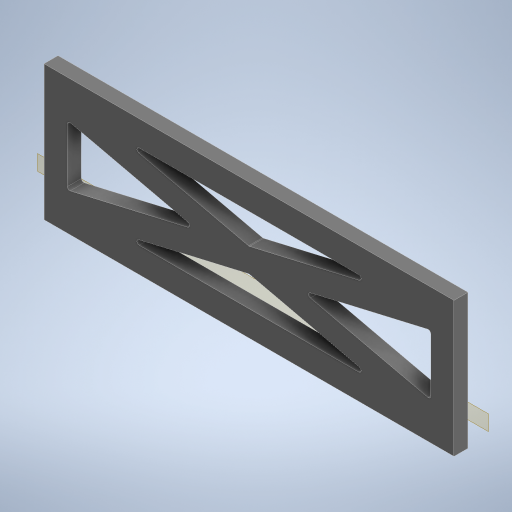
# Autodesk Inventor part: 13
Saved by Autodesk Inventor 2024.3 (Build 283343000, 343)
## iProperties
Created: 2024-09-08
Part Number: 13
Material: 아크릴, 선명
Document SubType Name: Modeling
Designer: 구지현
Density: 1.19 g/cm^3
Appearance: 회색
Mass: 52.1703 g
Surface Area: 217.666 cm^2
Volume: 43.8406 cm^3
Author: 구지현
Autodesk Inventor part; units mm, degrees
ref_plane "YZ Plane" through (0, 0, 0) normal (1, 0, 0) x (0, 1, 0)
ref_plane "XZ Plane" through (0, 0, 0) normal (0, 1, 0) x (-1, 0, 0)
ref_plane "XY Plane" through (0, 0, 0) normal (0, 0, 1) x (1, 0, 0)
ref_plane "작업 평면1" through (0, 0, 0) normal (0, 0, 1) x (1, 0, 0)
sketch "스케치1" plane through (0, 0, 0) normal (0, 0, 1) x (1, 0, 0)
  line L0 (0, 0) -> (176, 0) projected
  line L1 (176, 0) -> (176, 6) projected
  line L2 (0, 6) -> (176, 6) projected
  line L3 (0, 0) -> (0, 6) projected
  line L4 (0, 0) -> (176, 0)
  line L5 (176, 0) -> (176, 70)
  line L6 (176, 70) -> (0, 70)
  line L7 (0, 70) -> (0, 0)
  line L8 (0, 3) -> (25, 3)
  line L9 (25, 3) -> (25, 3)
  line L10 (25, 3) -> (0, 3)
  line L11 (0, 3) -> (0, 3)
  line L12 (25, 3) -> (67, 3)
  line L13 (67, 3) -> (109, 3)
  line L14 (109, 3) -> (151, 3)
  line L15 (151, 3) -> (176, 3)
  line L16 (151, 3) -> (151, 6)
  line L17 (151, 3) -> (151, 0)
  line L18 (109, 3) -> (109, 0)
  line L19 (109, 3) -> (109, 6)
  line L20 (67, 3) -> (67, 0)
  line L21 (67, 3) -> (67, 6)
  line L22 (25, 3) -> (25, 0)
  line L23 (25, 3) -> (25, 6)
  line L24 (0, 70) -> (0, 64)
  line L25 (0, 64) -> (176, 64)
  line L26 (25, 3) -> (25, 70)
  line L27 (67, 3) -> (67, 70)
  line L28 (109, 3) -> (109, 70)
  line L29 (151, 3) -> (151, 70)
  line L30 (20, 50) -> (156, 50)
  line L31 (156, 50) -> (156, 20)
  line L32 (156, 20) -> (18.9212, 20)
  line L33 (20, 50) -> (20, 20)
  point P0 (25, 0)
  point P1 (67, 0)
  point P2 (109, 0)
  point P3 (151, 0)
  point P4 (151, 64)
  point P5 (109, 64)
  point P6 (67, 64)
  point P7 (25, 64)
  point P8 (20, 38.5106)
  point P9 (76.3623, 50)
  point P10 (156, 43.8012)
  point P11 (88, 20)
  point P12 (151, 50)
  point P13 (151, 20)
  dimension "d0" = 176
  dimension "d1" = 70
  dimension "d2" = 25
  dimension "d3" = 42
  dimension "d4" = 42
  dimension "d5" = 42
  dimension "d6" = 25
  dimension "d7" = 6
  dimension "d10" = 20
  dimension "d11" = 20
  dimension "d12" = 20
  dimension "d13" = 20
  constraints: 60 end point, 22 point on line, 14 perpendicular, 5 equal length, 4 horizontal
  measures "d0" distance of L6.end L5.end
  measures "d1" distance of L5.end L4.end
  measures "d2" distance of L10.end L9.end
  measures "d3" distance of L8.end L12.end
  measures "d4" distance of L12.end L13.end
  measures "d5" distance of L13.end L14.end
  measures "d6" distance of L14.end L15.end
  measures "d7" distance of L6.end L24.end
  measures "d10" distance from line of L5 point (156, 43.801)
  measures "d11" distance from line of L6 point (76.362, 50)
  measures "d12" distance from line of L0 point (88, 20)
  measures "d13" distance from line of L7 point (20, 38.511)
extrude "돌출1" add sketch "스케치1" along normal blind 6 contours L3 L8 L22 L0 | L3 L2 L23 L8 | L20 L13 L18 L0 | L7 L25 L26 L30 L33 L32 L2 | L21 L2 L19 L13 | L26 L32 L27 L2 | L7 L6 L26 L25 | L17 L15 L1 L0 | L27 L32 L28 L2 | L25 L27 L30 L26 | L16 L2 L1 L15 | L28 L32 L29 L2 | L27 L6 L28 L25 | L25 L28 L30 L27 | L29 L32 L31 L30 L25 L5 L2 | L25 L29 L30 L28 | L29 L30 L31 L32 | L29 L6 L5 L25
move faces "이동1" translate (0, -10, 0) faces at (20, 30, 2) (107.3333, 20, 4) (151, 40, 4) (123, 6, 2) (159.3333, 0, 2) (81, 0, 4) (39, 6, 4) (8.3333, 0, 2) (25, 1, 2) (25, 4, 2) (109, 1, 2) (109, 4, 2) (67, 5, 2) (67, 2, 2) (151, 2, 2) (151, 5, 2)
sketch "스케치2" plane through (176, 70, 6) normal (1, 0, 0) x (0, 0, -1)
  line L0 (6, -60) -> (6, -74) projected
  line L1 (6, -74) -> (15, -74) projected
  line L2 (15, -74) -> (15, -80) projected
  line L3 (15, -80) -> (35, -80) projected
  line L4 (35, -80) -> (35, -74) projected
  line L5 (35, -74) -> (50, -74) projected
  line L6 (50, -74) -> (50, -80) projected
  line L7 (50, -80) -> (70, -80) projected
  line L8 (70, -80) -> (70, -74) projected
  line L9 (70, -74) -> (79, -74) projected
  line L10 (79, -74) -> (79, -60) projected
  line L11 (79, -60) -> (85, -60) projected
  line L12 (85, -60) -> (85, -20) projected
  line L13 (85, -20) -> (79, -20) projected
  line L14 (79, -20) -> (79, 0) projected
  line L15 (79, 0) -> (70, 0) projected
  line L16 (70, 0) -> (70, -6) projected
  line L17 (70, -6) -> (50, -6) projected
  line L18 (50, -6) -> (50, 0) projected
  line L19 (50, 0) -> (35, 0) projected
  line L20 (35, 0) -> (35, -6) projected
  line L21 (35, -6) -> (15, -6) projected
  line L22 (15, -6) -> (15, 0) projected
  line L23 (15, 0) -> (6, 0) projected
  line L24 (6, 0) -> (6, -20) projected
  line L25 (6, -20) -> (0, -20) projected
  line L26 (0, -20) -> (0, -60) projected
  line L27 (0, -60) -> (6, -60) projected
  line L28 (6, -80) -> (6, 0) projected
  line L29 (6, 0) -> (0, 0) projected
  line L30 (0, -80) -> (0, 0) projected
  line L31 (6, -80) -> (0, -80) projected
  point P0 (6, -70)
  point P1 (0, -60)
  point P2 (6, 0)
  point P3 (0, -20)
extrude "돌출2" cut sketch "스케치2" against normal blind 6 contours L28 L24 L23 L22 L21 L20 L19 L18 L17 L16 L15 L14 L13 L12 L11 L10 L9 L8 L7 L6 L5 L4 L3 L2 L1 L0 | L27 L26 L25 L28
sketch "스케치3" plane through (0, 70, 0) normal (-1, 0, 0) x (0, 0, 1)
  ellipse E0 centre (-18.9548, -43.9) end of major axis (-18.9548, -42.45) minor radius 1.45 projected
  ellipse E1 centre (-53.5548, -21.9) end of major axis (-53.5548, -20.45) minor radius 1.45 projected
  ellipse E2 centre (-18.9548, -65.9) end of major axis (-18.9548, -64.45) minor radius 1.45 projected
  circle A0 centre (-18.9548, -21.9) radius 1.45 projected
  circle A1 centre (-53.5548, -43.9) radius 1.45 projected
  ellipse E3 centre (-53.5548, -65.9) end of major axis (-53.5548, -64.45) minor radius 1.45 projected
  line L0 (-51.1548, -74) -> (-44, -74) projected
  line L1 (-44, -74) -> (-44, -80) projected
  line L2 (-44, -80) -> (-64, -80) projected
  line L3 (-64, -80) -> (-64, -74) projected
  line L4 (-64, -74) -> (-73, -74) projected
  line L5 (-73, -74) -> (-73, -60) projected
  line L6 (-73, -60) -> (-79, -60) projected
  line L7 (-79, -60) -> (-79, -20) projected
  line L8 (-79, -20) -> (-73, -20) projected
  line L9 (-73, -20) -> (-73, 0) projected
  line L10 (-73, 0) -> (-64, 0) projected
  line L11 (-64, 0) -> (-64, -6) projected
  line L12 (-64, -6) -> (-44, -6) projected
  line L13 (-44, -6) -> (-44, 0) projected
  line L14 (-44, 0) -> (-29, 0) projected
  line L15 (-29, 0) -> (-29, -6) projected
  line L16 (-29, -6) -> (-9, -6) projected
  line L17 (-9, -6) -> (-9, 0) projected
  line L18 (-9, 0) -> (0, 0) projected
  line L19 (0, 0) -> (0, -20) projected
  line L20 (0, -20) -> (6, -20) projected
  line L21 (6, -20) -> (6, -60) projected
  line L22 (6, -60) -> (0, -60) projected
  line L23 (0, -60) -> (0, -74) projected
  line L24 (0, -74) -> (-9, -74) projected
  line L25 (-9, -74) -> (-9, -80) projected
  line L26 (-9, -80) -> (-29, -80) projected
  line L27 (-29, -80) -> (-29, -74) projected
  line L28 (-29, -74) -> (-21.3548, -74) projected
  line L29 (-21.3548, -74) -> (-21.3548, -12.9525) projected
  line L30 (-21.3548, -12.9525) -> (-24.7548, -13) projected
  line L31 (-24.7548, -13) -> (-50.8207, -13) projected
  ellipse E4 centre (-50.1962, -14.9) end of major axis (-50.1962, -12.9) minor radius 2 (-50.8207, -13) -> (-50.8548, -13.0115) ccw projected
  line L32 (-50.8548, -13.0115) -> (-50.8548, -13) projected
  line L33 (-50.8548, -13) -> (-51.1548, -13) projected
  line L34 (-51.1548, -13) -> (-51.1548, -13.1447) projected
  ellipse E5 centre (-50.1962, -14.9) end of major axis (-50.1962, -16.9) minor radius 2 (-50.8548, -13.0115) -> (-51.1548, -13.1447) ccw projected
  line L35 (-50.8548, -13.0115) -> (-50.8548, -13.1178) projected
  arc A2 (-50.8548, -13.1178) -> (-51.1548, -13.2595) centre (-50.1963, -14.8999) ccw projected
  line L36 (-51.1548, -13.2595) -> (-51.1548, -74) projected
  line L37 (0, 0) -> (0, -80) projected
  line L38 (0, -80) -> (6, -80) projected
  line L39 (6, 0) -> (6, -80) projected
  line L40 (0, 0) -> (6, 0) projected
  point P0 (0, -70)
  point P1 (0, -20)
  point P2 (0, -60)
  constraints: 2 other
extrude "돌출3" cut sketch "스케치3" against normal blind 6 contours L37 L20 L21 L22
sketch "스케치4" plane through (0, 0, 6) normal (0, 0, 1) x (1, 0, 0)
  line L0 (54, 56) -> (20, 56) projected
  line L1 (20, 56) -> (20, 50) projected
  line L2 (20, 50) -> (54, 50) projected
  line L3 (54, 50) -> (54, 56) projected
  line L4 (117, 50) -> (151, 50) projected
  line L5 (151, 50) -> (151, 56) projected
  line L6 (151, 56) -> (117, 56) projected
  line L7 (117, 56) -> (117, 50) projected
  line L8 (117, 4) -> (151, 4) projected
  line L9 (151, 4) -> (151, 10) projected
  line L10 (151, 10) -> (117, 10) projected
  line L11 (117, 10) -> (117, 4) projected
  line L12 (54, 10) -> (20, 10) projected
  line L13 (20, 10) -> (20, 4) projected
  line L14 (20, 4) -> (54, 4) projected
  line L15 (54, 4) -> (54, 10) projected
  point P0 (0, 0)
extrude "돌출4" cut sketch "스케치4" against normal blind 6
sketch "스케치5" plane through (0, 0, 6) normal (0, 0, 1) x (1, 0, 0)
  line L0 (151, 56) -> (151, 10) projected
  line L1 (151, 10) -> (151, 4) projected
  line L2 (151, 4) -> (117, 4) projected
  line L3 (117, 4) -> (117, 10) projected
  line L4 (117, 10) -> (54, 10) projected
  line L5 (54, 10) -> (54, 4) projected
  line L6 (54, 4) -> (20, 4) projected
  line L7 (20, 4) -> (20, 56) projected
  line L8 (20, 56) -> (54, 56) projected
  line L9 (54, 56) -> (54, 50) projected
  line L10 (54, 50) -> (117, 50) projected
  line L11 (117, 50) -> (117, 56) projected
  line L12 (117, 56) -> (151, 56) projected
  line L13 (6, 10) -> (0, 10) projected
  line L14 (0, 10) -> (0, -10) projected
  line L15 (0, -10) -> (25, -10) projected
  line L16 (25, -10) -> (25, -4) projected
  line L17 (25, -4) -> (67, -4) projected
  line L18 (67, -4) -> (67, -10) projected
  line L19 (67, -10) -> (109, -10) projected
  line L20 (109, -10) -> (109, -4) projected
  line L21 (109, -4) -> (151, -4) projected
  line L22 (151, -4) -> (151, -10) projected
  line L23 (151, -10) -> (176, -10) projected
  line L24 (176, -10) -> (176, 10) projected
  line L25 (176, 10) -> (170, 10) projected
  line L26 (170, 10) -> (170, 50) projected
  line L27 (170, 50) -> (176, 50) projected
  line L28 (176, 50) -> (176, 70) projected
  line L29 (176, 70) -> (151, 70) projected
  line L30 (151, 70) -> (151, 64) projected
  line L31 (151, 64) -> (109, 64) projected
  line L32 (109, 64) -> (109, 70) projected
  line L33 (109, 70) -> (67, 70) projected
  line L34 (67, 70) -> (67, 64) projected
  line L35 (67, 64) -> (25, 64) projected
  line L36 (25, 64) -> (25, 70) projected
  line L37 (25, 70) -> (0, 70) projected
  line L38 (0, 70) -> (0, 50) projected
  line L39 (0, 50) -> (6, 50) projected
  line L40 (6, 50) -> (6, 10) projected
  line L41 (0, 70) -> (176, 70)
  line L42 (176, 70) -> (176, -10)
  line L43 (176, -10) -> (0, -10)
  line L44 (0, -10) -> (0, 70)
  point P0 (0, 0)
  point P1 (176, 50)
  point P2 (0, 10)
  point P3 (67, 70)
  constraints: 8 end point, 2 parallel, 1 horizontal, 1 perpendicular
extrude "돌출5" add sketch "스케치5" against normal up to surface (6 mm away) contours L0 L1 L2 L3 L4 L5 L6 L7 L8 L9 L10 L11 L12 | L13 L44 L39 L40 | L16 L17 L18 L43 | L41 L34 L35 L36 | L20 L21 L22 L43 | L41 L30 L31 L32 | L25 L26 L27 L42
sketch "스케치6" plane through (0, 0, 6) normal (0, 0, 1) x (1, 0, 0)
  line L0 (0, 70) -> (0, -10) projected
  line L1 (0, -10) -> (176, -10) projected
  line L2 (176, -10) -> (176, 70) projected
  line L3 (176, 70) -> (0, 70) projected
  line L4 (166, 0) -> (10, 0)
  line L5 (10, 0) -> (10, 60)
  line L6 (10, 60) -> (166, 60)
  line L7 (166, 60) -> (166, 0)
  line L8 (10, 60) -> (166, 0)
  line L9 (10, 0) -> (166, 60)
  line L10 (11.4359, 63.7334) -> (167.4359, 3.7334)
  line L11 (8.5641, 3.7334) -> (164.5641, 63.7334)
  line L12 (11.4359, -3.7334) -> (167.4359, 56.2666)
  line L13 (8.5641, 56.2666) -> (164.5641, -3.7334)
  point P0 (0, 0)
  point P1 (154.8573, 0)
  point P2 (88, 25.7143)
  point P3 (21.1427, 0)
  point P4 (166, 55.7143)
  point P5 (99.1427, 30)
  point P6 (166, 4.2857)
  point P7 (88, 34.2857)
  point P8 (154.8573, 60)
  point P9 (21.1427, 60)
  point P10 (76.8573, 30)
  point P11 (10, 55.7143)
  point P12 (10, 4.2857)
  dimension "d25" = 10
  dimension "d26" = 4
  dimension "d27" = 4
  dimension "d28" = 4
  dimension "d29" = 4
  constraints: 20 end point, 4 parallel, 3 other
  measures "d25" distance between parallel lines of L1 L4
  measures "d26" distance between parallel lines of L8 L10
  measures "d27" distance between parallel lines of L9 L11
  measures "d28" distance between parallel lines of L9 L12
  measures "d29" distance between parallel lines of L8 L13
extrude "돌출6" cut sketch "스케치6" against normal through all contours L4 L12 L13 | L10 L12 L7 | L5 L13 L11 | L11 L10 L6
fillet "모깎기1" radius 5 11 edges at (10, 55.7143, 3) (21.1427, 60, 3) (154.8573, 60, 3) (166, 55.7143, 3) (166, 4.2857, 3) (99.1427, 30, 3) (88, 34.2857, 3) (76.8573, 30, 3) (88, 25.7143, 3) (10, 4.2857, 3) (21.1427, 0, 3)
sketch "스케치7" plane through (0, 0, 0) normal (0, 0, -1) x (-1, 0, 0)
  line L0 (-166, 11.5658) -> (-166, 48.4342) projected
  arc A0 (-159.2051, 53.1009) -> (-166, 48.4342) centre (-161, 48.4342) ccw projected
  line L1 (-159.2051, 53.1009) -> (-111.2762, 34.6667) projected
  arc A1 (-111.2762, 25.3333) -> (-111.2762, 34.6667) centre (-113.0711, 30) ccw projected
  line L2 (-111.2762, 25.3333) -> (-159.2051, 6.8991) projected
  arc A2 (-166, 11.5658) -> (-159.2051, 6.8991) centre (-161, 11.5658) ccw projected
  line L3 (-46.2762, 50.3333) -> (-86.2051, 34.976) projected
  arc A3 (-89.7949, 34.976) -> (-86.2051, 34.976) centre (-88, 39.6427) ccw projected
  line L4 (-89.7949, 34.976) -> (-129.7238, 50.3333) projected
  arc A4 (-127.9289, 60) -> (-129.7238, 50.3333) centre (-127.9289, 55) ccw projected
  line L5 (-127.9289, 60) -> (-48.0711, 60) projected
  arc A5 (-46.2762, 50.3333) -> (-48.0711, 60) centre (-48.0711, 55) ccw projected
  line L6 (-48.0711, 0) -> (-154.8573, 0) projected
  line L7 (-154.8573, 0) -> (-89.7949, 25.024) projected
  arc A6 (-86.2051, 25.024) -> (-89.7949, 25.024) centre (-88, 20.3573) ccw projected
  line L8 (-86.2051, 25.024) -> (-46.2762, 9.6667) projected
  arc A7 (-48.0711, 0) -> (-46.2762, 9.6667) centre (-48.0711, 5) ccw projected
  line L9 (-16.7949, 6.8991) -> (-64.7238, 25.3333) projected
  arc A8 (-64.7238, 34.6667) -> (-64.7238, 25.3333) centre (-62.9289, 30) ccw projected
  line L10 (-64.7238, 34.6667) -> (-16.7949, 53.1009) projected
  arc A9 (-10, 48.4342) -> (-16.7949, 53.1009) centre (-15, 48.4342) ccw projected
  line L11 (-10, 48.4342) -> (-10, 11.5658) projected
  arc A10 (-16.7949, 6.8991) -> (-10, 11.5658) centre (-15, 11.5658) ccw projected
  line L12 (-176, 70) -> (0, 70) projected
  line L13 (-176, -10) -> (-176, 70) projected
  line L14 (0, -10) -> (-176, -10) projected
  line L15 (0, 70) -> (0, -10) projected
  point P0 (0, 0)
extrude "돌출7" add sketch "스케치7" against normal blind 6 contours L0 A0 L1 A1 L2 A2 | L3 A3 L4 A4 L5 A5 | L6 L7 A6 L8 A7 | L9 A8 L10 A9 L11 A10
sketch "스케치8" plane through (0, 0, 0) normal (0, 0, -1) x (-1, 0, 0)
  line L0 (-171.5, 41.2) -> (-173.5, 41.2) projected
  line L1 (-171.5, 46.2) -> (-173.5, 46.2)
  line L2 (-176, 70) -> (0, 70) projected
  line L3 (-176, -10) -> (-176, 70) projected
  line L4 (0, -10) -> (-176, -10) projected
  line L5 (0, 70) -> (0, -10) projected
  line L6 (-176, -10) -> (0, -10)
  line L7 (0, -10) -> (0, 46.2)
  line L8 (0, 46.2) -> (-176, 46.2)
  line L9 (-176, 46.2) -> (-176, -10)
  point P0 (0, 0)
  dimension "d35" = 5
  constraints: 10 end point, 4 equal length, 1 perpendicular
  measures "d35" distance between parallel lines of L0 L1
extrude "돌출8" cut sketch "스케치8" against normal through all contours L1 L8 L3 L2 L5
sketch "스케치9" plane through (0, 0, 0) normal (0, 0, -1) x (-1, 0, 0)
  line L0 (0, 46.2) -> (-176, 46.2) projected
  line L1 (-176, -10) -> (-176, 46.2) projected
  line L2 (0, -10) -> (-176, -10) projected
  line L3 (0, 46.2) -> (0, -10) projected
  line L4 (-166, 36.2) -> (-10, 36.2)
  line L5 (-10, 36.2) -> (-10, 0)
  line L6 (-10, 0) -> (-166, 0)
  line L7 (-166, 0) -> (-166, 36.2)
  line L8 (-166, 36.2) -> (-10, 0)
  line L9 (-166, 0) -> (-10, 36.2)
  line L10 (-164.8698, 41.0706) -> (-8.8698, 4.8706)
  line L11 (-167.1302, 4.8706) -> (-11.1302, 41.0706)
  line L12 (-164.8698, -4.8706) -> (-8.8698, 31.3294)
  line L13 (-167.1302, 31.3294) -> (-11.1302, -4.8706)
  point P0 (0, 0)
  point P1 (-32.1195, 0)
  point P2 (-88, 12.9671)
  point P3 (-143.8805, 0)
  point P4 (-10, 31.0671)
  point P5 (-65.8805, 18.1)
  point P6 (-10, 5.1329)
  point P7 (-88, 23.2329)
  point P8 (-32.1195, 36.2)
  point P9 (-143.8805, 36.2)
  point P10 (-110.1195, 18.1)
  point P11 (-166, 31.0671)
  point P12 (-166, 5.1329)
  dimension "d38" = 10
  dimension "d39" = 5
  dimension "d40" = 5
  dimension "d41" = 5
  dimension "d42" = 5
  constraints: 20 end point, 4 parallel, 3 other
  measures "d38" distance between parallel lines of L0 L4
  measures "d39" distance between parallel lines of L8 L10
  measures "d40" distance between parallel lines of L9 L11
  measures "d41" distance between parallel lines of L9 L12
  measures "d42" distance between parallel lines of L8 L13
extrude "돌출9" cut sketch "스케치9" against normal through all contours L4 L11 L10 | L13 L11 L7 | L5 L10 L12 | L12 L13 L6
fillet "모깎기2" radius 1 12 edges at (166, 5.1329, 3) (166, 31.0671, 3) (110.1195, 18.1, 3) (143.8805, 36.2, 3) (88, 23.2329, 3) (32.1195, 36.2, 3) (65.8805, 18.1, 3) (10, 31.0671, 3) (10, 5.1329, 3) (32.1195, 0, 3) (88, 12.9671, 3) (143.8805, 0, 3)
sketch "스케치10" plane through (0, 0, 0) normal (0, 0, -1) x (-1, 0, 0)
  line L0 (-10, 29.8085) -> (-10, 6.3915) projected
  arc A0 (-11.226, 5.4174) -> (-10, 6.3915) centre (-11, 6.3915) ccw projected
  line L1 (-11.226, 5.4174) -> (-61.6827, 17.1259) projected
  arc A1 (-61.6827, 19.0741) -> (-61.6827, 17.1259) centre (-61.4566, 18.1) ccw projected
  line L2 (-61.6827, 19.0741) -> (-11.226, 30.7826) projected
  arc A2 (-10, 29.8085) -> (-11.226, 30.7826) centre (-11, 29.8085) ccw projected
  line L3 (-88.226, 23.2853) -> (-135.3733, 34.2259) projected
  arc A3 (-135.1472, 36.2) -> (-135.3733, 34.2259) centre (-135.1472, 35.2) ccw projected
  line L4 (-135.1472, 36.2) -> (-40.8528, 36.2) projected
  arc A4 (-40.6267, 34.2259) -> (-40.8528, 36.2) centre (-40.8528, 35.2) ccw projected
  line L5 (-40.6267, 34.2259) -> (-87.774, 23.2853) projected
  arc A5 (-88.226, 23.2853) -> (-87.774, 23.2853) centre (-88, 24.2594) ccw projected
  line L6 (-40.8528, 0) -> (-135.1472, 0) projected
  arc A6 (-135.3733, 1.9741) -> (-135.1472, 0) centre (-135.1472, 1) ccw projected
  line L7 (-135.3733, 1.9741) -> (-88.226, 12.9147) projected
  arc A7 (-87.774, 12.9147) -> (-88.226, 12.9147) centre (-88, 11.9406) ccw projected
  line L8 (-87.774, 12.9147) -> (-40.6267, 1.9741) projected
  arc A8 (-40.8528, 0) -> (-40.6267, 1.9741) centre (-40.8528, 1) ccw projected
  line L9 (-114.3173, 17.1259) -> (-164.774, 5.4174) projected
  arc A9 (-166, 6.3915) -> (-164.774, 5.4174) centre (-165, 6.3915) ccw projected
  line L10 (-166, 6.3915) -> (-166, 29.8085) projected
  arc A10 (-164.774, 30.7826) -> (-166, 29.8085) centre (-165, 29.8085) ccw projected
  line L11 (-164.774, 30.7826) -> (-114.3173, 19.0741) projected
  arc A11 (-114.3173, 17.1259) -> (-114.3173, 19.0741) centre (-114.5434, 18.1) ccw projected
  line L12 (0, 46.2) -> (-176, 46.2) projected
  line L13 (-176, -10) -> (-176, 46.2) projected
  line L14 (0, -10) -> (-176, -10) projected
  line L15 (0, 46.2) -> (0, -10) projected
  line L16 (-176, -10.9) -> (0, -10.9)
  line L17 (0, -10.9) -> (0, 47.1)
  line L18 (0, 47.1) -> (-176, 47.1)
  line L19 (-176, 47.1) -> (-176, -10.9)
  line L20 (-176, -10.9) -> (0, 47.1) construction
  line L21 (0, -10.9) -> (-176, 47.1) construction
  point P0 (0, 0)
  point P1 (-88, 18.1)
  point P2 (-176, 46.2)
  dimension "d46" = 176
  dimension "d47" = 58
  constraints: 12 end point, 2 midpoint, 2 parallel, 1 horizontal, 1 perpendicular
  measures "d46" distance of L18.end L17.end
  measures "d47" distance of L17.end L16.end
extrude "돌출10" add sketch "스케치10" against normal up to surface (6 mm away) contours L12 L19 L18 L17 | L17 L16 L19 L14
